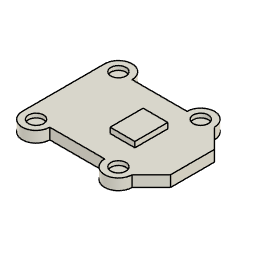
colour_sensor_cover (Autodesk Fusion 360 design; units mm, degrees)
part number: 2025-08-25-11-06-01-160
Autodesk Fusion 360 part; units mm, degrees
note: some values were not read from the file. Set by a fixed rule: which sketch regions a step uses.
sketch "Colour Sensor Cover" plane through (0, 0, 0) normal (0, 0, 1) x (1, 0, 0)
  line L0 (0, 0) -> (47, 0)
  line L1 (47, 0) -> (47, 30)
  line L2 (47, 30) -> (0, 30)
  line L3 (0, 30) -> (0, 0)
  circle A0 centre (5, 30) radius 5
  circle A1 centre (35, 30) radius 5
  circle A2 centre (5, 0) radius 5
  circle A3 centre (35, 0) radius 5
  dimension "d1" = 47
  dimension "d2" = 30
  dimension "d3" = 10
  dimension "d4" = 10
  dimension "d5" = 10
  dimension "d6" = 10
  dimension "d7" = 5
  dimension "d8" = 5
  dimension "d9" = 12
  dimension "d10" = 12
  constraint horizontal L0
  constraint vertical L1
  constraint horizontal L2
  constraint vertical L3
  constraint coincident L0.start L3.end
  constraint coincident L2 A0.centre
  constraint coincident L2 A1.centre
  constraint coincident L0 A2.centre
  constraint coincident L0 A3.centre
  measures "d1" distance of L0.start L0.end
  measures "d2" distance of L0.end L1.end
  measures "d3" diameter of A0
  measures "d4" diameter of A1
  measures "d5" diameter of A2
  measures "d6" diameter of A3
  measures "d7" distance of L2.end A0.centre
  measures "d8" distance of L0.start A2.centre
  measures "d9" distance of L1.end A1.centre
  measures "d10" distance of L0.end A3.centre
extrude "Extrude1" add sketch "Colour Sensor Cover" along normal blind 4
chamfer "Chamfer1" distance 7 angle 45 2 edges at (47, 0, 2) (47, 30, 2)
sketch "Magnet Holes" plane through (0, 0, 4) normal (0, 0, 1) x (-1, 0, 0)
  line L0 (-47, -23) -> (-40, -30)
  arc A0 (-40, -30) -> (-30, -30) centre (-35, -30) ccw
  line L1 (-30, -30) -> (-10, -30)
  arc A1 (-10, -30) -> (0, -30) centre (-5, -30) ccw
  line L2 (0, -30) -> (0, 0)
  arc A2 (0, 0) -> (-10, 0) centre (-5, 0) ccw
  line L3 (-10, 0) -> (-30, 0)
  arc A3 (-30, 0) -> (-40, 0) centre (-35, 0) ccw
  line L4 (-40, 0) -> (-47, -7)
  line L5 (-47, -7) -> (-47, -23)
  circle A4 centre (-5, -30) radius 2.75
  circle A5 centre (-35, -30) radius 2.75
  circle A6 centre (-5, 0) radius 2.75
  circle A7 centre (-35, 0) radius 2.75
  dimension "d14" = 5.5
  dimension "d15" = 5.5
  dimension "d16" = 5.5
  dimension "d17" = 5.5
  constraint concentric A1 A4
  constraint concentric A0 A5
  constraint concentric A2 A6
  constraint concentric A3 A7
  measures "d14" diameter of A4
  measures "d15" diameter of A5
  measures "d16" diameter of A6
  measures "d17" diameter of A7
extrude "Extrude2" cut sketch "Magnet Holes" against normal blind 1.5 contours A4 | A5 | A6 | A7
sketch "Colour Sensor Support" plane through (0, 0, 4) normal (0, 0, 1) x (-1, 0, 0)
  circle A0 centre (-5, -30) radius 2.75
  circle A1 centre (-35, -30) radius 2.75
  circle A2 centre (-5, 0) radius 2.75
  circle A3 centre (-35, 0) radius 2.75
  line L0 (-47, -23) -> (-40, -30)
  arc A4 (-40, -30) -> (-30, -30) centre (-35, -30) ccw
  line L1 (-30, -30) -> (-10, -30)
  arc A5 (-10, -30) -> (0, -30) centre (-5, -30) ccw
  line L2 (0, -30) -> (0, 0)
  arc A6 (0, 0) -> (-10, 0) centre (-5, 0) ccw
  line L3 (-10, 0) -> (-30, 0)
  arc A7 (-30, 0) -> (-40, 0) centre (-35, 0) ccw
  line L4 (-40, 0) -> (-47, -7)
  line L5 (-47, -7) -> (-47, -23)
  line L6 (-23, -21) -> (-32, -21)
  line L7 (-32, -21) -> (-32, -9)
  line L8 (-32, -9) -> (-23, -9)
  line L9 (-23, -9) -> (-23, -21)
  dimension "d20" = 9
  dimension "d21" = 9
  dimension "d22" = 15
  dimension "d23" = 9
  dimension "d24" = 12
  constraint horizontal L6
  constraint vertical L7
  constraint horizontal L8
  constraint vertical L9
  measures "d20" distance of L1 L6
  measures "d21" distance of L3 L8
  measures "d22" distance of L5 L7
  measures "d23" distance of L6.start L6.end
  measures "d24" distance of L6.end L7.end
extrude "Extrude3" add sketch "Colour Sensor Support" along normal blind 2 contours L6 L7 L8 L9
equation "d9 = 7 mm + 5 mm"
equation "d10 = 7 mm + 5 mm"
named bodies: "Colour Sensor Cover"
